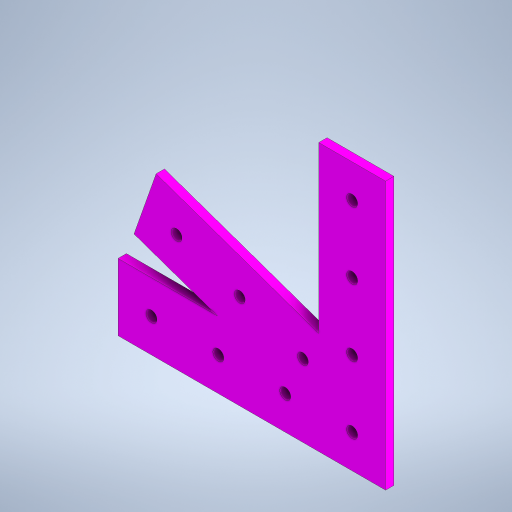
# Autodesk Inventor part: arrow bracket (70.1 and 19.29 degrees)
Saved by Autodesk Inventor 2023 (Build 270158030, 158C)
## iProperties
Created: 2022-07-22
Part Number: arrow bracket (70.1 and 19.29 degrees)
Material: Generic
Document SubType Name: Modeling
Designer: kt1040502
Density: 1 g/cm^3
Appearance: Default
Author: kt1040502
Autodesk Inventor part; units mm, degrees
ref_plane "YZ Plane" through (0, 0, 0) normal (1, 0, 0) x (0, 1, 0)
ref_plane "XZ Plane" through (0, 0, 0) normal (0, 1, 0) x (-1, 0, 0)
ref_plane "Work Plane1" through (0, 0, 0) normal (0, 0, 1) x (1, 0, 0)
sketch "Sketch1" plane through (0, 0, 0) normal (0, 0, 1) x (1, 0, 0)
  line L0 (-533.4, -800.8554) -> (-63.844, -965.2) projected
  line L1 (-533.4, -965.2) -> (-25.4, -965.2) projected
  line L2 (-25.4, -951.7446) -> (-494.956, -787.4) projected
  line L3 (-533.4, -990.6) -> (-25.4, -990.6) projected
  line L4 (-25.4, -787.4) -> (-25.4, -1498.6) projected
  line L5 (0, -787.4) -> (0, -1498.6) projected
  arc A0 (-40.1687, -977.9762) -> (-36.0313, -977.9762) centre (-38.1, -977.9) ccw projected
  arc A1 (-36.0313, -977.8238) -> (-40.1687, -977.8238) centre (-38.1, -977.9) ccw projected
  arc A2 (-65.5687, -977.9762) -> (-61.4313, -977.9762) centre (-63.5, -977.9) ccw projected
  arc A3 (-61.4313, -977.8238) -> (-65.5687, -977.8238) centre (-63.5, -977.9) ccw projected
  line L6 (-116.3687, -977.8238) -> (-137.6313, -977.8238) projected
  arc A4 (-12.7762, -975.8313) -> (-12.7762, -979.9687) centre (-12.7, -977.9) ccw projected
  arc A5 (-12.6238, -979.9687) -> (-12.6238, -975.8313) centre (-12.7, -977.9) ccw projected
  arc A6 (-12.7762, -950.4313) -> (-12.7762, -954.5687) centre (-12.7, -952.5) ccw projected
  arc A7 (-12.6238, -954.5687) -> (-12.6238, -950.4313) centre (-12.7, -952.5) ccw projected
  arc A8 (-12.7762, -925.0313) -> (-12.7762, -929.1687) centre (-12.7, -927.1) ccw projected
  arc A9 (-12.6238, -929.1687) -> (-12.6238, -925.0313) centre (-12.7, -927.1) ccw projected
  circle A10 centre (-31.3935, -963.1023) radius 2.032 projected
  circle A11 centre (-55.3675, -954.7114) radius 2.032 projected
  circle A12 centre (-79.3415, -946.3205) radius 2.032 projected
  arc A13 (-12.7762, -899.6313) -> (-12.7762, -903.7687) centre (-12.7, -901.7) ccw projected
  arc A14 (-12.6238, -903.7687) -> (-12.6238, -899.6313) centre (-12.7, -901.7) ccw projected
  arc A15 (-90.9687, -977.9762) -> (-86.8313, -977.9762) centre (-88.9, -977.9) ccw projected
  arc A16 (-86.8313, -977.8238) -> (-90.9687, -977.8238) centre (-88.9, -977.9) ccw projected
  line L7 (-12.7, -901.7) -> (-12.7, -876.3) construction
  line L8 (-25.4, -889) -> (0, -889) construction
  line L9 (0, -889) -> (-25.4, -889)
  line L10 (-88.9, -977.9) -> (-114.3, -977.9) construction
  line L11 (-101.6, -990.6) -> (-101.6, -965.2)
  line L12 (-101.6, -990.6) -> (0, -990.6)
  line L13 (0, -990.6) -> (0, -889)
  line L14 (-25.4, -889) -> (-25.4, -951.7446)
  line L15 (-101.6, -965.2) -> (-63.844, -965.2)
  line L16 (-79.3415, -946.3205) -> (-103.3155, -937.9296) construction
  line L17 (-95.524, -954.112) -> (-87.1331, -930.138) construction
  line L18 (-87.1331, -930.138) -> (-95.524, -954.112)
  line L19 (-95.524, -954.112) -> (-63.844, -965.2)
  line L20 (-87.1331, -930.138) -> (-25.4, -951.7446)
  circle A17 centre (-12.7, -901.7) radius 2.0701
  circle A18 centre (-12.7, -927.1) radius 2.0701
  circle A19 centre (-12.7, -952.5) radius 2.0701
  circle A20 centre (-12.7, -977.9) radius 2.0701
  circle A21 centre (-38.1, -977.9) radius 2.0701
  circle A22 centre (-63.5, -977.9) radius 2.0701
  circle A23 centre (-88.9, -977.9) radius 2.0701
  circle A24 centre (-79.3415, -946.3205) radius 2.032
  circle A25 centre (-55.3675, -954.7114) radius 2.032
  circle A26 centre (-31.3935, -963.1023) radius 2.032
  point P0 (0, 0)
  point P1 (-12.7762, -903.7687)
  point P2 (-12.6238, -899.6313)
  point P3 (-12.7762, -929.1687)
  point P4 (-12.6238, -925.0313)
  point P5 (-12.7762, -954.5687)
  point P6 (-12.6238, -950.4313)
  point P7 (-12.7762, -979.9687)
  point P8 (-12.6238, -975.8313)
  point P9 (-86.8313, -977.9762)
  point P10 (-40.1687, -977.8238)
  point P11 (-36.0313, -977.9762)
  point P12 (-25.4, -990.6)
  dimension "d0" = 25.4
  dimension "d1" = 25.4
  dimension "d2" = 25.4
  constraints: 28 end point, 10 centre point, 10 coincident, 10 concentric, 8 point on line, 6 perpendicular, 2 collinear, 2 parallel, 1 horizontal, 1 vertical
  measures "d0" distance of L7.start L7.end
  measures "d1" distance of L10.start L10.end
  measures "d2" distance of L16.start L16.end
extrude "Extrusion1" add sketch "Sketch1" along normal blind 3.175
body "Solid1"
